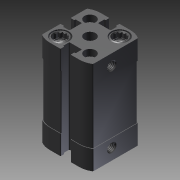
# Autodesk Inventor part: 536203 ADN-15-P---(Z)
Saved by Autodesk Inventor 2011 SP1 (Build 150282100, 282)
## iProperties
Created: 2018-05-28
Part Number: 536203 ADN-15-P---(Z)
Catalog Web Link: www.cadenas.de
Description: ADN-(Z)-Compact cylinder - Z
Vendor: FESTO
Document SubType Name: Modeling
Designer: psAdmin
Manufacturer: FESTO
Mass: 25.558 g
Surface Area: 133.612 cm^2
Volume: 25.558 cm^3
Density: 1 g/cm^3
Category: PARTsolutions
Company: FESTO
Title: 536203 ADN-15-P---(Z)
Author: Cadenas PARTsolutions
Comments: Compact cylinder - Z
PSOL_IDENT_0: {$CADENAS_DATA\23d-libs\festo\parts\a\adn\parts\adn_zr.prj},210 {VTYP=3D},{NB=536203 ADN-15-P---(Z)}
PSOL_IDENT_1: ,{LINA=536203 ADN-15-P---(Z)},{NN=ADN-(Z)},{DATE=06.10.2015 11:54:02},{GEOMDATE=22.09.2015 09:31:00}
PSOL_IDENT_2: ,{VERSION=},{LINEID=5510},{LINESUBID=-1},{WBVAR=HUB,DF,Q,S2S20,S1,R8,TT}  {NB=536203 ADN-15-P---(Z)}
PSOL_IDENT_3: ,{LINA=536203 ADN-15-P---(Z)},{KT=536203},{TNR=536203},{AUSF=ADN},{KDM=12},{BG=17.000},{VERS=1},{HUB
PSOL_IDENT_4: P=-},{HUB=15.00000},{HUB1=[1-300]},{HUB2=-},{HUB3=0},{THC='A','I'},{DF=P},{GA=A},{HUBL=variable},{HU
PSOL_IDENT_5: BC=hubc error},{Q=-},{VAR1C='-','Q'},{S2S20=-},{VAR2C='-','S2'},{VAR5C='-','S6'},{S1=-},{R8=-},{R81='
PSOL_IDENT_6: -'},{TT=-},{TT1='-'},{VAR6C='-'},{VAR7C='-','R3'},{HUBALG=[1-300]},{A=10.000},{A1=0.000},{AF=8.000},
PSOL_IDENT_7: {AF1=0.000},{AF2=8.000},{AF3=0.000},{B=0.000},{B1=0.000},{BG1=0.000},{D1=9.000},{D2=6.000},{D3=32.00
PSOL_IDENT_8: 0},{D4=0.000},{D5=4.000},{D6=M3},{D7=3.000},{D8=0.000},{D9=0.000},{E=27.500},{EE=M5},{EEN=5.000},{EE
PSOL_IDENT_9: 1=-},{J=10.500},{J1=2.000},{J11=2},{J2=0.000},{KF=4-48 UNF-2B},{KF1=-},{KF2=4-45 UNF-2B},{KF3=-},{KK=
PSOL_IDENT_10: 10-32 UNF-2A},{KK1=-},{L1=1.500},{L2=35.000},{L3=2.100},{L4=3.500},{L5=0.000},{L6=46.000},{L7=12.000
PSOL_IDENT_11: },{L8=0.000},{L9=1.500},{L10=0.000},{L11=0.000},{MF=6.000},{MM=6.000},{MM1=0.000},{PL=6.000},{RT=M4}
PSOL_IDENT_12: ,{RTN=4},{RTNK=3.242},{SF=3/16},{SF1=-},{SW=5.500},{TG=16.000},{VD=0.000},{VD1=0.000},{WH=4.200},{WH
PSOL_IDENT_13: 1=0.000},{WL=2.700},{WL1=0.000},{Y1=0.300},{Y2=0.500},{ZJ=39.200},{ZM=43.400},{RU=16.600},{R1=10.350
PSOL_IDENT_14: },{R2=0.600},{RA=0.600},{RB1=5.400},{RB2=6.800},{RT1=3.400},{DSK=6.000},{MDK=5.500},{MK=3.000},{MT=1
PSOL_IDENT_15: .300},{MS=2.500},{RUB=0.200},{KFN=3.000},{KFK=2.459},{B111=9.200},{B11=1.000},{B2=5.000},{B3=8.500},
PSOL_IDENT_16: {B4=3.500},{B5=3.000},{B6=6.000},{B7=17.000},{B8=4.000},{B9=6.000},{B10=7.200},{W=0.400},{S=6.000},{
PSOL_IDENT_17: LA=0.000},{LA1=0.000},{LA2=5.500},{LA3=7.000},{LA31=8.000},{LA4=0.000},{LA5=0.000},{LA6=0.000},{RR=4
PSOL_IDENT_18: .000},{LA7=0.000},{LA8=0.000},{LA9=0.000},{LA10=0.000},{ES=0.000},{SS=0.000},{TS=0.000},{WS=0.000},{
PSOL_IDENT_19: DK=0.000},{KS=0.000},{QN=},{S2N=},{S1S20N=},{R8N=},{TTN=},{DFALG='P'}
NN: ADN-(Z)
NT: Compact cylinder - Z
NB: 536203 ADN-15-P---(Z)
NBSYN: $TNR. $AUSF.-$HUB.-$DF.$QN.$S2N.$S1S20N.$R8N.$TTN.---(Z)
LINA: 536203 ADN-15-P---(Z)
TNR: 536203
AUSF: ADN
KDM: 12
BG: 17.000
HUB: 15.00000
DF: P
GA: A
Q: -
S2S20: -
S1: -
R8: -
TT: -
A: 10.000
A1: 0.000
AF: 8.000
AF1: 0.000
AF2: 8.000
AF3: 0.000
B: 0.000
B1: 0.000
BG1: 0.000
D1: 9.000
D2: 6.000
D3: 32.000
D4: 0.000
D5: 4.000
D6: M3
D7: 3.000
D8: 0.000
D9: 0.000
E: 27.500
EE: M5
EE1: -
J: 10.500
J1: 2.000
J2: 0.000
KF: 4-48 UNF-2B
KF1: -
KF2: 4-45 UNF-2B
KF3: -
KK: 10-32 UNF-2A
KK1: -
L1: 1.500
L2: 35.000
L3: 2.100
L4: 3.500
L5: 0.000
L6: 46.000
L7: 12.000
L8: 0.000
L9: 1.500
L10: 0.000
L11: 0.000
MF: 6.000
MM: 6.000
MM1: 0.000
PL: 6.000
RT: M4
RTNK: 3.242
SF: 3/16
SF1: -
SW: 5.500
TG: 16.000
VD: 0.000
VD1: 0.000
WH: 4.200
WH1: 0.000
WL: 2.700
WL1: 0.000
Y1: 0.300
Y2: 0.500
ZJ: 39.200
ZM: 43.400
RU: 16.600
R1: 10.350
R2: 0.600
RA: 0.600
DSK: 6.000
MDK: 5.500
MK: 3.000
MT: 1.300
MS: 2.500
RUB: 0.200
B111: 9.200
B11: 1.000
B2: 5.000
B3: 8.500
B4: 3.500
B5: 3.000
B6: 6.000
B7: 17.000
B8: 4.000
B9: 6.000
B10: 7.200
W: 0.400
S: 6.000
LA: 0.000
LA1: 0.000
LA2: 5.500
LA3: 7.000
LA31: 8.000
LA4: 0.000
LA5: 0.000
LA6: 0.000
RR: 4.000
LA7: 0.000
LA8: 0.000
LA9: 0.000
LA10: 0.000
ES: 0.000
SS: 0.000
TS: 0.000
WS: 0.000
DK: 0.000
KS: 0.000
SUPPLIER: FESTO
ARTICLENO: 536203 ADN-15-P---(Z)
BOMINFO: 536203 ADN-15-P---(Z)
CREATOR: CADENAS GmbH
Autodesk Inventor part; units mm, degrees
sketch "Sketch_26" plane through (0, 0, 0) normal (0, 0, 1) x (1, 0, 0)
  line L0 (-13.75, -2.5) -> (-13.75, -11.5793)
  arc A0 (-13.75, -11.5793) -> (-13.3272, -12.3141) centre (-12.9, -11.5793) ccw
  arc A1 (-13.3272, -12.3141) -> (-8, -13.75) centre (-8, -3.15) ccw
  line L1 (-8, -13.75) -> (-2.5, -13.75)
  arc A2 (-2.5, -13.75) -> (-2.1, -13.35) centre (-2.5, -13.35) ccw
  line L2 (-2.1, -13.35) -> (-2.1, -11.9)
  arc A3 (-2.1, -11.9) -> (-2.3, -11.7) centre (-2.3, -11.9) ccw
  line L3 (-2.3, -11.7) -> (-2.6, -11.7)
  arc A4 (-2.8, -11.5) -> (-2.6, -11.7) centre (-2.6, -11.5) ccw
  line L4 (-2.8, -11.5) -> (-2.8, -8.7)
  arc A5 (-2.4, -8.3) -> (-2.8, -8.7) centre (-2.4, -8.7) ccw
  line L5 (-2.4, -8.3) -> (3.6, -8.3)
  arc A6 (4, -8.7) -> (3.6, -8.3) centre (3.6, -8.7) ccw
  line L6 (4, -8.7) -> (4, -11.5)
  arc A7 (3.8, -11.7) -> (4, -11.5) centre (3.8, -11.5) ccw
  line L7 (3.8, -11.7) -> (3.5, -11.7)
  arc A8 (3.5, -11.7) -> (3.3, -11.9) centre (3.5, -11.9) ccw
  line L8 (3.3, -11.9) -> (3.3, -13.35)
  arc A9 (3.3, -13.35) -> (3.7, -13.75) centre (3.7, -13.35) ccw
  line L9 (3.7, -13.75) -> (8, -13.75)
  arc A10 (8, -13.75) -> (13.3272, -12.3141) centre (8, -3.15) ccw
  arc A11 (13.3272, -12.3141) -> (13.75, -11.5793) centre (12.9, -11.5793) ccw
  line L10 (13.75, -11.5793) -> (13.75, 11.5793)
  arc A12 (13.75, 11.5793) -> (13.3272, 12.3141) centre (12.9, 11.5793) ccw
  arc A13 (13.3272, 12.3141) -> (8, 13.75) centre (8, 3.15) ccw
  line L11 (8, 13.75) -> (2.5, 13.75)
  arc A14 (2.5, 13.75) -> (2.1, 13.35) centre (2.5, 13.35) ccw
  line L12 (2.1, 13.35) -> (2.1, 11.9)
  arc A15 (2.1, 11.9) -> (2.3, 11.7) centre (2.3, 11.9) ccw
  line L13 (2.3, 11.7) -> (2.6, 11.7)
  arc A16 (2.8, 11.5) -> (2.6, 11.7) centre (2.6, 11.5) ccw
  line L14 (2.8, 11.5) -> (2.8, 8.7)
  arc A17 (2.4, 8.3) -> (2.8, 8.7) centre (2.4, 8.7) ccw
  line L15 (2.4, 8.3) -> (-3.6, 8.3)
  arc A18 (-4, 8.7) -> (-3.6, 8.3) centre (-3.6, 8.7) ccw
  line L16 (-4, 8.7) -> (-4, 11.5)
  arc A19 (-3.8, 11.7) -> (-4, 11.5) centre (-3.8, 11.5) ccw
  line L17 (-3.8, 11.7) -> (-3.5, 11.7)
  arc A20 (-3.5, 11.7) -> (-3.3, 11.9) centre (-3.5, 11.9) ccw
  line L18 (-3.3, 11.9) -> (-3.3, 13.35)
  arc A21 (-3.3, 13.35) -> (-3.7, 13.75) centre (-3.7, 13.35) ccw
  line L19 (-3.7, 13.75) -> (-8, 13.75)
  arc A22 (-8, 13.75) -> (-13.3272, 12.3141) centre (-8, 3.15) ccw
  arc A23 (-13.3272, 12.3141) -> (-13.75, 11.5793) centre (-12.9, 11.5793) ccw
  line L20 (-13.75, 11.5793) -> (-13.75, 3.7)
  arc A24 (-13.75, 3.7) -> (-13.35, 3.3) centre (-13.35, 3.7) ccw
  line L21 (-13.35, 3.3) -> (-11.9, 3.3)
  arc A25 (-11.9, 3.3) -> (-11.7, 3.5) centre (-11.9, 3.5) ccw
  line L22 (-11.7, 3.5) -> (-11.7, 3.8)
  arc A26 (-11.5, 4) -> (-11.7, 3.8) centre (-11.5, 3.8) ccw
  line L23 (-11.5, 4) -> (-8.7, 4)
  arc A27 (-8.3, 3.6) -> (-8.7, 4) centre (-8.7, 3.6) ccw
  line L24 (-8.3, 3.6) -> (-8.3, -2.4)
  arc A28 (-8.7, -2.8) -> (-8.3, -2.4) centre (-8.7, -2.4) ccw
  line L25 (-8.7, -2.8) -> (-11.5, -2.8)
  arc A29 (-11.7, -2.6) -> (-11.5, -2.8) centre (-11.5, -2.6) ccw
  line L26 (-11.7, -2.6) -> (-11.7, -2.3)
  arc A30 (-11.7, -2.3) -> (-11.9, -2.1) centre (-11.9, -2.3) ccw
  line L27 (-11.9, -2.1) -> (-13.35, -2.1)
  arc A31 (-13.35, -2.1) -> (-13.75, -2.5) centre (-13.35, -2.5) ccw
  constraints: 64 point on circle, 56 end point, 32 centre point
extrude "Extrusion1" add sketch "Sketch_26" against normal blind 50
sketch "Sketch_112" plane through (0, 0, -10.5) normal (0, 0, 1) x (1, 0, 0)
  line L0 (-27.5, -27.5) -> (27.5, -27.5)
  line L1 (27.5, -27.5) -> (27.5, 27.5)
  line L2 (27.5, 27.5) -> (-27.5, 27.5)
  line L3 (-27.5, 27.5) -> (-27.5, -27.5)
  line L4 (-13.5, -2.5) -> (-13.5, -11.3293)
  arc A0 (-13.5, -11.3293) -> (-13.0772, -12.0641) centre (-12.65, -11.3293) ccw
  arc A1 (-13.0772, -12.0641) -> (-7.75, -13.5) centre (-7.75, -2.9) ccw
  line L5 (-7.75, -13.5) -> (-2.5, -13.5)
  arc A2 (-2.5, -13.5) -> (-2.1, -13.1) centre (-2.5, -13.1) ccw
  line L6 (-2.1, -13.1) -> (-2.1, -11.85)
  arc A3 (-2.1, -11.85) -> (-2.25, -11.7) centre (-2.25, -11.85) ccw
  line L7 (-2.25, -11.7) -> (-2.6, -11.7)
  arc A4 (-2.8, -11.5) -> (-2.6, -11.7) centre (-2.6, -11.5) ccw
  line L8 (-2.8, -11.5) -> (-2.8, -8.7)
  arc A5 (-2.4, -8.3) -> (-2.8, -8.7) centre (-2.4, -8.7) ccw
  line L9 (-2.4, -8.3) -> (3.6, -8.3)
  arc A6 (4, -8.7) -> (3.6, -8.3) centre (3.6, -8.7) ccw
  line L10 (4, -8.7) -> (4, -11.5)
  arc A7 (3.8, -11.7) -> (4, -11.5) centre (3.8, -11.5) ccw
  line L11 (3.8, -11.7) -> (3.45, -11.7)
  arc A8 (3.45, -11.7) -> (3.3, -11.85) centre (3.45, -11.85) ccw
  line L12 (3.3, -11.85) -> (3.3, -13.1)
  arc A9 (3.3, -13.1) -> (3.7, -13.5) centre (3.7, -13.1) ccw
  line L13 (3.7, -13.5) -> (7.75, -13.5)
  arc A10 (7.75, -13.5) -> (13.0772, -12.0641) centre (7.75, -2.9) ccw
  arc A11 (13.0772, -12.0641) -> (13.5, -11.3293) centre (12.65, -11.3293) ccw
  line L14 (13.5, -11.3293) -> (13.5, 11.3293)
  arc A12 (13.5, 11.3293) -> (13.0772, 12.0641) centre (12.65, 11.3293) ccw
  arc A13 (13.0772, 12.0641) -> (7.75, 13.5) centre (7.75, 2.9) ccw
  line L15 (7.75, 13.5) -> (2.5, 13.5)
  arc A14 (2.5, 13.5) -> (2.1, 13.1) centre (2.5, 13.1) ccw
  line L16 (2.1, 13.1) -> (2.1, 11.85)
  arc A15 (2.1, 11.85) -> (2.25, 11.7) centre (2.25, 11.85) ccw
  line L17 (2.25, 11.7) -> (2.6, 11.7)
  arc A16 (2.8, 11.5) -> (2.6, 11.7) centre (2.6, 11.5) ccw
  line L18 (2.8, 11.5) -> (2.8, 8.7)
  arc A17 (2.4, 8.3) -> (2.8, 8.7) centre (2.4, 8.7) ccw
  line L19 (2.4, 8.3) -> (-3.6, 8.3)
  arc A18 (-4, 8.7) -> (-3.6, 8.3) centre (-3.6, 8.7) ccw
  line L20 (-4, 8.7) -> (-4, 11.5)
  arc A19 (-3.8, 11.7) -> (-4, 11.5) centre (-3.8, 11.5) ccw
  line L21 (-3.8, 11.7) -> (-3.45, 11.7)
  arc A20 (-3.45, 11.7) -> (-3.3, 11.85) centre (-3.45, 11.85) ccw
  line L22 (-3.3, 11.85) -> (-3.3, 13.1)
  arc A21 (-3.3, 13.1) -> (-3.7, 13.5) centre (-3.7, 13.1) ccw
  line L23 (-3.7, 13.5) -> (-7.75, 13.5)
  arc A22 (-7.75, 13.5) -> (-13.0772, 12.0641) centre (-7.75, 2.9) ccw
  arc A23 (-13.0772, 12.0641) -> (-13.5, 11.3293) centre (-12.65, 11.3293) ccw
  line L24 (-13.5, 11.3293) -> (-13.5, 3.7)
  arc A24 (-13.5, 3.7) -> (-13.1, 3.3) centre (-13.1, 3.7) ccw
  line L25 (-13.1, 3.3) -> (-11.85, 3.3)
  arc A25 (-11.85, 3.3) -> (-11.7, 3.45) centre (-11.85, 3.45) ccw
  line L26 (-11.7, 3.45) -> (-11.7, 3.8)
  arc A26 (-11.5, 4) -> (-11.7, 3.8) centre (-11.5, 3.8) ccw
  line L27 (-11.5, 4) -> (-8.7, 4)
  arc A27 (-8.3, 3.6) -> (-8.7, 4) centre (-8.7, 3.6) ccw
  line L28 (-8.3, 3.6) -> (-8.3, -2.4)
  arc A28 (-8.7, -2.8) -> (-8.3, -2.4) centre (-8.7, -2.4) ccw
  line L29 (-8.7, -2.8) -> (-11.5, -2.8)
  arc A29 (-11.7, -2.6) -> (-11.5, -2.8) centre (-11.5, -2.6) ccw
  line L30 (-11.7, -2.6) -> (-11.7, -2.25)
  arc A30 (-11.7, -2.25) -> (-11.85, -2.1) centre (-11.85, -2.25) ccw
  line L31 (-11.85, -2.1) -> (-13.1, -2.1)
  arc A31 (-13.1, -2.1) -> (-13.5, -2.5) centre (-13.1, -2.5) ccw
  constraints: 64 end point, 64 point on circle, 32 centre point
extrude "Extrusion2" cut sketch "Sketch_112" against normal blind 29
sketch "Skizze_3_ALT_Drilling_1" plane through (0, -2, 0) normal (0, 1, 0) x (1, 0, 0)
  line L0 (13.75, 6) -> (6.75, 6)
  line L1 (6.75, 6) -> (6.75, 8.067)
  line L2 (6.75, 8.067) -> (13.317, 8.067)
  line L3 (13.317, 8.067) -> (13.75, 8.5)
  line L4 (13.75, 8.5) -> (13.75, 6)
  line L5 (13.75, 6) -> (6.75, 6)
  constraints: 12 end point
revolve "Revolution1" cut sketch "Skizze_3_ALT_Drilling_1" angle 360 about axis through (13.75, -2, -6) along (1, 0, 0)
thread "Thread1" size "M5x0.8" class "6H" standard "ISO Metric profile" length 5.067
sketch "Skizze_4_ALT_Drilling_2" plane through (0, -2, 0) normal (0, 1, 0) x (1, 0, 0)
  line L0 (13.75, 44) -> (5.75, 44)
  line L1 (5.75, 44) -> (5.75, 46.067)
  line L2 (5.75, 46.067) -> (13.317, 46.067)
  line L3 (13.317, 46.067) -> (13.75, 46.5)
  line L4 (13.75, 46.5) -> (13.75, 44)
  line L5 (13.75, 44) -> (5.75, 44)
  constraints: 12 end point
revolve "Revolution2" cut sketch "Skizze_4_ALT_Drilling_2" angle 360 about axis through (13.75, -2, -44) along (1, 0, 0)
thread "Thread2" size "M5x0.8" class "6H" standard "ISO Metric profile" length 5.067
sketch "Skizze_5_ALT_Drilling_3" plane through (0, 0, 0) normal (1, 0, 0) x (0, 1, 0)
  line L0 (0, -38) -> (0, 1)
  line L1 (0, 1) -> (3, 1)
  line L2 (3, 1) -> (3, -20)
  line L3 (3, -20) -> (6, -20)
  line L4 (6, -20) -> (6, -38)
  line L5 (6, -38) -> (0, -38)
  line L6 (0, -38) -> (0, 1)
  constraints: 14 end point
revolve "Revolution3" cut sketch "Skizze_5_ALT_Drilling_3" angle 360 about axis through (0, 0, -38) along (0, 0, -1)
sketch "Skizze_7_ALT_Drilling_4" plane through (0, 0, 0) normal (1, 0, 0) x (0, 1, 0)
  line L0 (0, -50) -> (0, -47.9)
  line L1 (0, -47.9) -> (4.5, -47.9)
  line L2 (4.5, -47.9) -> (4.5, -50)
  line L3 (4.5, -50) -> (0, -50)
  line L4 (0, -50) -> (0, -47.9)
  constraints: 10 end point
revolve "Revolution4" cut sketch "Skizze_7_ALT_Drilling_4" angle 360 about axis through (0, 0, -50) along (0, 0, -1)
sketch "Skizze_8_ALT_Drilling_5" plane through (8, 0, 0) normal (1, 0, 0) x (0, 0, -1)
  line L0 (17, 8) -> (0, 8)
  line L1 (0, 8) -> (0, 12.6)
  line L2 (0, 12.6) -> (5, 12.6)
  line L3 (5, 12.6) -> (5, 11)
  line L4 (5, 11) -> (17, 11)
  line L5 (17, 11) -> (17, 8)
  line L6 (17, 8) -> (0, 8)
  constraints: 14 end point
revolve "Revolution5" cut sketch "Skizze_8_ALT_Drilling_5" angle 360 about axis through (8, 8, -17) along (0, 0, -1)
sketch "Sketch_27" plane through (8, 0, 0) normal (1, 0, 0) x (0, 0, -1)
  line L0 (17, 8) -> (0, 8)
  line L1 (0, 11.6) -> (1.0392, 11)
  line L2 (1.0392, 11) -> (3.5, 11)
  line L3 (3.5, 11) -> (3.5, 10)
  line L4 (3.5, 10) -> (3.879, 9.621)
  line L5 (3.879, 9.621) -> (17, 9.621)
  line L6 (17, 9.621) -> (17, 12)
  line L7 (17, 12) -> (5, 12)
  line L8 (5, 12) -> (5, 12.25)
  line L9 (5, 12.25) -> (0.4, 12.25)
  line L10 (0.4, 12.25) -> (0, 11.85)
  line L11 (0, 11.85) -> (0, 11.6)
  constraints: 24 end point
revolve "Revolution6" add sketch "Sketch_27" angle 360 about axis through (8, 8, -17) along (0, 0, -1)
thread "Thread3" size "M4x0.7" class "6H" standard "ISO Metric profile" full length
sketch "Sketch_1_ALT_Drilling_6" plane through (8, 0, 0) normal (1, 0, 0) x (0, 0, -1)
  line L0 (50, 8) -> (33, 8)
  line L1 (33, 8) -> (33, 11)
  line L2 (33, 11) -> (45, 11)
  line L3 (45, 11) -> (45, 12.6)
  line L4 (45, 12.6) -> (50, 12.6)
  line L5 (50, 12.6) -> (50, 8)
  line L6 (50, 8) -> (33, 8)
  constraints: 14 end point
revolve "Revolution7" cut sketch "Sketch_1_ALT_Drilling_6" angle 360 about axis through (8, 8, -50) along (0, 0, -1)
sketch "Sketch_86_ALT_Drilling_7" plane through (8, 0, 0) normal (1, 0, 0) x (0, 0, -1)
  line L0 (33, 8) -> (17, 8)
  line L1 (17, 8) -> (17, 10)
  line L2 (17, 10) -> (33, 10)
  line L3 (33, 10) -> (33, 8)
  line L4 (33, 8) -> (17, 8)
  constraints: 10 end point
revolve "Revolution8" cut sketch "Sketch_86_ALT_Drilling_7" angle 360 about axis through (8, 8, -33) along (0, 0, -1)
sketch "Sketch_28" plane through (8, 0, 0) normal (1, 0, 0) x (0, 0, -1)
  line L0 (50, 8) -> (33, 8)
  line L1 (33, 12) -> (33, 9.621)
  line L2 (33, 9.621) -> (46.121, 9.621)
  line L3 (46.121, 9.621) -> (46.5, 10)
  line L4 (46.5, 10) -> (46.5, 11)
  line L5 (46.5, 11) -> (48.9608, 11)
  line L6 (48.9608, 11) -> (50, 11.6)
  line L7 (50, 11.6) -> (50, 11.85)
  line L8 (50, 11.85) -> (49.6, 12.25)
  line L9 (49.6, 12.25) -> (45, 12.25)
  line L10 (45, 12.25) -> (45, 12)
  line L11 (45, 12) -> (33, 12)
  constraints: 24 end point
revolve "Revolution9" add sketch "Sketch_28" angle 360 about axis through (8, 8, -50) along (0, 0, -1)
thread "Thread4" size "M4x0.7" class "6H" standard "ISO Metric profile" full length
sketch "Skizze_9_ALT_Drilling_8" plane through (-8, 0, 0) normal (1, 0, 0) x (0, 0, -1)
  line L0 (25, -8) -> (0, -8)
  line L1 (0, -8) -> (0, -3.4)
  line L2 (0, -3.4) -> (5, -3.4)
  line L3 (5, -3.4) -> (5, -5)
  line L4 (5, -5) -> (17, -5)
  line L5 (17, -5) -> (17, -8)
  line L6 (17, -8) -> (0, -8)
  constraints: 14 end point
revolve "Revolution10" cut sketch "Skizze_9_ALT_Drilling_8" angle 360 about axis through (-8, -8, -25) along (0, 0, -1)
sketch "Sketch_2_ALT_Drilling_9" plane through (-8, 0, 0) normal (1, 0, 0) x (0, 0, -1)
  line L0 (50, -8) -> (33, -8)
  line L1 (33, -8) -> (33, -5)
  line L2 (33, -5) -> (45, -5)
  line L3 (45, -5) -> (45, -3.4)
  line L4 (45, -3.4) -> (50, -3.4)
  line L5 (50, -3.4) -> (50, -8)
  line L6 (50, -8) -> (33, -8)
  constraints: 14 end point
revolve "Revolution11" cut sketch "Sketch_2_ALT_Drilling_9" angle 360 about axis through (-8, -8, -50) along (0, 0, -1)
sketch "Sketch_29" plane through (-8, 0, 0) normal (1, 0, 0) x (0, 0, -1)
  line L0 (17, -8) -> (0, -8)
  line L1 (0, -4.4) -> (1.0392, -5)
  line L2 (1.0392, -5) -> (3.5, -5)
  line L3 (3.5, -5) -> (3.5, -6)
  line L4 (3.5, -6) -> (3.879, -6.379)
  line L5 (3.879, -6.379) -> (17, -6.379)
  line L6 (17, -6.379) -> (17, -4)
  line L7 (17, -4) -> (5, -4)
  line L8 (5, -4) -> (5, -3.75)
  line L9 (5, -3.75) -> (0.4, -3.75)
  line L10 (0.4, -3.75) -> (0, -4.15)
  line L11 (0, -4.15) -> (0, -4.4)
  constraints: 24 end point
revolve "Revolution12" add sketch "Sketch_29" angle 360 about axis through (-8, -8, -17) along (0, 0, -1)
thread "Thread5" size "M4x0.7" class "6H" standard "ISO Metric profile" full length
sketch "Sketch_30" plane through (-8, 0, 0) normal (1, 0, 0) x (0, 0, -1)
  line L0 (50, -8) -> (33, -8)
  line L1 (33, -4) -> (33, -6.379)
  line L2 (33, -6.379) -> (46.121, -6.379)
  line L3 (46.121, -6.379) -> (46.5, -6)
  line L4 (46.5, -6) -> (46.5, -5)
  line L5 (46.5, -5) -> (48.9608, -5)
  line L6 (48.9608, -5) -> (50, -4.4)
  line L7 (50, -4.4) -> (50, -4.15)
  line L8 (50, -4.15) -> (49.6, -3.75)
  line L9 (49.6, -3.75) -> (45, -3.75)
  line L10 (45, -3.75) -> (45, -4)
  line L11 (45, -4) -> (33, -4)
  constraints: 24 end point
revolve "Revolution13" add sketch "Sketch_30" angle 360 about axis through (-8, -8, -50) along (0, 0, -1)
thread "Thread6" size "M4x0.7" class "6H" standard "ISO Metric profile" full length
sketch "Skizze_12_ALT_Drilling_10" plane through (8, 0, 0) normal (1, 0, 0) x (0, 0, -1)
  line L0 (33, -8) -> (-0.1, -8)
  line L1 (-0.1, -8) -> (-0.1, -5)
  line L2 (-0.1, -5) -> (3.5, -5)
  line L3 (3.5, -5) -> (3.5, -6)
  line L4 (3.5, -6) -> (3.879, -6.379)
  line L5 (3.879, -6.379) -> (33, -6.379)
  line L6 (33, -6.379) -> (33, -8)
  line L7 (33, -8) -> (-0.1, -8)
  constraints: 16 end point
revolve "Revolution14" cut sketch "Skizze_12_ALT_Drilling_10" angle 360 about axis through (8, -8, -33) along (0, 0, -1)
thread "Thread7" size "M4x0.7" class "6H" standard "ISO Metric profile" length 6.621
sketch "Sketch_123" plane through (8, 0, 0) normal (1, 0, 0) x (0, 0, -1)
  line L0 (33, -8) -> (10.5, -8)
  line L1 (10.5, -8) -> (10.5, -4)
  line L2 (10.5, -4) -> (33, -4)
  line L3 (33, -4) -> (33, -8)
  line L4 (33, -8) -> (10.5, -8)
  constraints: 10 end point
revolve "Revolution15" add sketch "Sketch_123" angle 360 about axis through (8, -8, -33) along (0, 0, -1)
sketch "Sketch_124_ALT_Drilling_11" plane through (8, 0, 0) normal (1, 0, 0) x (0, 0, -1)
  line L0 (33, -8) -> (10.5, -8)
  line L1 (10.5, -8) -> (10.5, -6)
  line L2 (10.5, -6) -> (33, -6)
  line L3 (33, -6) -> (33, -8)
  line L4 (33, -8) -> (10.5, -8)
  constraints: 10 end point
revolve "Revolution16" cut sketch "Sketch_124_ALT_Drilling_11" angle 360 about axis through (8, -8, -33) along (0, 0, -1)
sketch "Sketch_3_ALT_Drilling_12" plane through (8, 0, 0) normal (1, 0, 0) x (0, 0, -1)
  line L0 (50.1, -8) -> (25, -8)
  line L1 (25, -8) -> (25, -6.379)
  line L2 (25, -6.379) -> (46.121, -6.379)
  line L3 (46.121, -6.379) -> (46.5, -6)
  line L4 (46.5, -6) -> (46.5, -5)
  line L5 (46.5, -5) -> (50.1, -5)
  line L6 (50.1, -5) -> (50.1, -8)
  line L7 (50.1, -8) -> (25, -8)
  constraints: 16 end point
revolve "Revolution17" cut sketch "Sketch_3_ALT_Drilling_12" angle 360 about axis through (8, -8, -50.1) along (0, 0, -1)
thread "Thread8" size "M4x0.7" class "6H" standard "ISO Metric profile" length 6.621
sketch "Sketch_117" plane through (8, 0, 0) normal (1, 0, 0) x (0, 0, -1)
  line L0 (39.5, -8) -> (17, -8)
  line L1 (17, -8) -> (17, -4)
  line L2 (17, -4) -> (39.5, -4)
  line L3 (39.5, -4) -> (39.5, -8)
  line L4 (39.5, -8) -> (17, -8)
  constraints: 10 end point
revolve "Revolution18" add sketch "Sketch_117" angle 360 about axis through (8, -8, -39.5) along (0, 0, -1)
sketch "Sketch_119_ALT_Drilling_13" plane through (8, 0, 0) normal (1, 0, 0) x (0, 0, -1)
  line L0 (39.5, -8) -> (17, -8)
  line L1 (17, -8) -> (17, -6)
  line L2 (17, -6) -> (39.5, -6)
  line L3 (39.5, -6) -> (39.5, -8)
  line L4 (39.5, -8) -> (17, -8)
  constraints: 10 end point
revolve "Revolution19" cut sketch "Sketch_119_ALT_Drilling_13" angle 360 about axis through (8, -8, -39.5) along (0, 0, -1)
sketch "Skizze_13_ALT_Drilling_14" plane through (-8, 0, 0) normal (1, 0, 0) x (0, 0, -1)
  line L0 (33, 8) -> (-0.1, 8)
  line L1 (-0.1, 8) -> (-0.1, 11)
  line L2 (-0.1, 11) -> (3.5, 11)
  line L3 (3.5, 11) -> (3.5, 10)
  line L4 (3.5, 10) -> (3.879, 9.621)
  line L5 (3.879, 9.621) -> (33, 9.621)
  line L6 (33, 9.621) -> (33, 8)
  line L7 (33, 8) -> (-0.1, 8)
  constraints: 16 end point
revolve "Revolution20" cut sketch "Skizze_13_ALT_Drilling_14" angle 360 about axis through (-8, 8, -33) along (0, 0, -1)
thread "Thread9" size "M4x0.7" class "6H" standard "ISO Metric profile" length 6.621
sketch "Sketch_121" plane through (-8, 0, 0) normal (1, 0, 0) x (0, 0, -1)
  line L0 (33, 8) -> (10.5, 8)
  line L1 (10.5, 8) -> (10.5, 12)
  line L2 (10.5, 12) -> (33, 12)
  line L3 (33, 12) -> (33, 8)
  line L4 (33, 8) -> (10.5, 8)
  constraints: 10 end point
revolve "Revolution21" add sketch "Sketch_121" angle 360 about axis through (-8, 8, -33) along (0, 0, -1)
sketch "Sketch_122_ALT_Drilling_15" plane through (-8, 0, 0) normal (1, 0, 0) x (0, 0, -1)
  line L0 (33, 8) -> (10.5, 8)
  line L1 (10.5, 8) -> (10.5, 10)
  line L2 (10.5, 10) -> (33, 10)
  line L3 (33, 10) -> (33, 8)
  line L4 (33, 8) -> (10.5, 8)
  constraints: 10 end point
revolve "Revolution22" cut sketch "Sketch_122_ALT_Drilling_15" angle 360 about axis through (-8, 8, -33) along (0, 0, -1)
sketch "Sketch_4_ALT_Drilling_16" plane through (-8, 0, 0) normal (1, 0, 0) x (0, 0, -1)
  line L0 (50.1, 8) -> (25, 8)
  line L1 (25, 8) -> (25, 9.621)
  line L2 (25, 9.621) -> (46.121, 9.621)
  line L3 (46.121, 9.621) -> (46.5, 10)
  line L4 (46.5, 10) -> (46.5, 11)
  line L5 (46.5, 11) -> (50.1, 11)
  line L6 (50.1, 11) -> (50.1, 8)
  line L7 (50.1, 8) -> (25, 8)
  constraints: 16 end point
revolve "Revolution23" cut sketch "Sketch_4_ALT_Drilling_16" angle 360 about axis through (-8, 8, -50.1) along (0, 0, -1)
thread "Thread10" size "M4x0.7" class "6H" standard "ISO Metric profile" length 6.621
sketch "Sketch_118" plane through (-8, 0, 0) normal (1, 0, 0) x (0, 0, -1)
  line L0 (39.5, 8) -> (17, 8)
  line L1 (17, 8) -> (17, 12)
  line L2 (17, 12) -> (39.5, 12)
  line L3 (39.5, 12) -> (39.5, 8)
  line L4 (39.5, 8) -> (17, 8)
  constraints: 10 end point
revolve "Revolution24" add sketch "Sketch_118" angle 360 about axis through (-8, 8, -39.5) along (0, 0, -1)
sketch "Sketch_120_ALT_Drilling_17" plane through (-8, 0, 0) normal (1, 0, 0) x (0, 0, -1)
  line L0 (39.5, 8) -> (17, 8)
  line L1 (17, 8) -> (17, 10)
  line L2 (17, 10) -> (39.5, 10)
  line L3 (39.5, 10) -> (39.5, 8)
  line L4 (39.5, 8) -> (17, 8)
  constraints: 10 end point
revolve "Revolution25" cut sketch "Sketch_120_ALT_Drilling_17" angle 360 about axis through (-8, 8, -39.5) along (0, 0, -1)
sketch "Sketch_85_ALT_Drilling_18" plane through (-8, 0, 0) normal (1, 0, 0) x (0, 0, -1)
  line L0 (33, -8) -> (17, -8)
  line L1 (17, -8) -> (17, -6)
  line L2 (17, -6) -> (33, -6)
  line L3 (33, -6) -> (33, -8)
  line L4 (33, -8) -> (17, -8)
  constraints: 10 end point
revolve "Revolution26" cut sketch "Sketch_85_ALT_Drilling_18" angle 360 about axis through (-8, -8, -33) along (0, 0, -1)
sketch "Sketch_8" plane through (0, 0, 0) normal (0, 0, 1) x (1, 0, 0)
  line L0 (-11.4641, -8) -> (-11, -8.8038)
  line L1 (-11, -8.8038) -> (-11, -9.7321)
  line L2 (-11, -9.7321) -> (-10.1962, -10.1962)
  line L3 (-10.1962, -10.1962) -> (-9.7321, -11)
  line L4 (-9.7321, -11) -> (-8.8038, -11)
  line L5 (-8.8038, -11) -> (-8, -11.4641)
  line L6 (-8, -11.4641) -> (-7.1962, -11)
  line L7 (-7.1962, -11) -> (-6.2679, -11)
  line L8 (-6.2679, -11) -> (-5.8038, -10.1962)
  line L9 (-5.8038, -10.1962) -> (-5, -9.7321)
  line L10 (-5, -9.7321) -> (-5, -8.8038)
  line L11 (-5, -8.8038) -> (-4.5359, -8)
  line L12 (-4.5359, -8) -> (-5, -7.1962)
  line L13 (-5, -7.1962) -> (-5, -6.2679)
  line L14 (-5, -6.2679) -> (-5.8038, -5.8038)
  line L15 (-5.8038, -5.8038) -> (-6.2679, -5)
  line L16 (-6.2679, -5) -> (-7.1962, -5)
  line L17 (-7.1962, -5) -> (-8, -4.5359)
  line L18 (-8, -4.5359) -> (-8.8038, -5)
  line L19 (-8.8038, -5) -> (-9.7321, -5)
  line L20 (-9.7321, -5) -> (-10.1962, -5.8038)
  line L21 (-10.1962, -5.8038) -> (-11, -6.2679)
  line L22 (-11, -6.2679) -> (-11, -7.1962)
  line L23 (-11, -7.1962) -> (-11.4641, -8)
  constraints: 48 end point
extrude "Extrusion3" cut sketch "Sketch_8" against normal blind 3
sketch "Sketch_7" plane through (0, 0, 0) normal (0, 0, 1) x (1, 0, 0)
  line L0 (4.5359, 8) -> (5, 7.1962)
  line L1 (5, 7.1962) -> (5, 6.2679)
  line L2 (5, 6.2679) -> (5.8038, 5.8038)
  line L3 (5.8038, 5.8038) -> (6.2679, 5)
  line L4 (6.2679, 5) -> (7.1962, 5)
  line L5 (7.1962, 5) -> (8, 4.5359)
  line L6 (8, 4.5359) -> (8.8038, 5)
  line L7 (8.8038, 5) -> (9.7321, 5)
  line L8 (9.7321, 5) -> (10.1962, 5.8038)
  line L9 (10.1962, 5.8038) -> (11, 6.2679)
  line L10 (11, 6.2679) -> (11, 7.1962)
  line L11 (11, 7.1962) -> (11.4641, 8)
  line L12 (11.4641, 8) -> (11, 8.8038)
  line L13 (11, 8.8038) -> (11, 9.7321)
  line L14 (11, 9.7321) -> (10.1962, 10.1962)
  line L15 (10.1962, 10.1962) -> (9.7321, 11)
  line L16 (9.7321, 11) -> (8.8038, 11)
  line L17 (8.8038, 11) -> (8, 11.4641)
  line L18 (8, 11.4641) -> (7.1962, 11)
  line L19 (7.1962, 11) -> (6.2679, 11)
  line L20 (6.2679, 11) -> (5.8038, 10.1962)
  line L21 (5.8038, 10.1962) -> (5, 9.7321)
  line L22 (5, 9.7321) -> (5, 8.8038)
  line L23 (5, 8.8038) -> (4.5359, 8)
  constraints: 48 end point
extrude "Extrusion4" cut sketch "Sketch_7" against normal blind 3
sketch "Sketch_9" plane through (0, 0, -50) normal (0, 0, 1) x (1, 0, 0)
  line L0 (-11.4641, -8) -> (-11, -8.8038)
  line L1 (-11, -8.8038) -> (-11, -9.7321)
  line L2 (-11, -9.7321) -> (-10.1962, -10.1962)
  line L3 (-10.1962, -10.1962) -> (-9.7321, -11)
  line L4 (-9.7321, -11) -> (-8.8038, -11)
  line L5 (-8.8038, -11) -> (-8, -11.4641)
  line L6 (-8, -11.4641) -> (-7.1962, -11)
  line L7 (-7.1962, -11) -> (-6.2679, -11)
  line L8 (-6.2679, -11) -> (-5.8038, -10.1962)
  line L9 (-5.8038, -10.1962) -> (-5, -9.7321)
  line L10 (-5, -9.7321) -> (-5, -8.8038)
  line L11 (-5, -8.8038) -> (-4.5359, -8)
  line L12 (-4.5359, -8) -> (-5, -7.1962)
  line L13 (-5, -7.1962) -> (-5, -6.2679)
  line L14 (-5, -6.2679) -> (-5.8038, -5.8038)
  line L15 (-5.8038, -5.8038) -> (-6.2679, -5)
  line L16 (-6.2679, -5) -> (-7.1962, -5)
  line L17 (-7.1962, -5) -> (-8, -4.5359)
  line L18 (-8, -4.5359) -> (-8.8038, -5)
  line L19 (-8.8038, -5) -> (-9.7321, -5)
  line L20 (-9.7321, -5) -> (-10.1962, -5.8038)
  line L21 (-10.1962, -5.8038) -> (-11, -6.2679)
  line L22 (-11, -6.2679) -> (-11, -7.1962)
  line L23 (-11, -7.1962) -> (-11.4641, -8)
  constraints: 48 end point
extrude "Extrusion5" cut sketch "Sketch_9" along normal blind 3
sketch "Sketch_10" plane through (0, 0, -50) normal (0, 0, 1) x (1, 0, 0)
  line L0 (4.5359, 8) -> (5, 7.1962)
  line L1 (5, 7.1962) -> (5, 6.2679)
  line L2 (5, 6.2679) -> (5.8038, 5.8038)
  line L3 (5.8038, 5.8038) -> (6.2679, 5)
  line L4 (6.2679, 5) -> (7.1962, 5)
  line L5 (7.1962, 5) -> (8, 4.5359)
  line L6 (8, 4.5359) -> (8.8038, 5)
  line L7 (8.8038, 5) -> (9.7321, 5)
  line L8 (9.7321, 5) -> (10.1962, 5.8038)
  line L9 (10.1962, 5.8038) -> (11, 6.2679)
  line L10 (11, 6.2679) -> (11, 7.1962)
  line L11 (11, 7.1962) -> (11.4641, 8)
  line L12 (11.4641, 8) -> (11, 8.8038)
  line L13 (11, 8.8038) -> (11, 9.7321)
  line L14 (11, 9.7321) -> (10.1962, 10.1962)
  line L15 (10.1962, 10.1962) -> (9.7321, 11)
  line L16 (9.7321, 11) -> (8.8038, 11)
  line L17 (8.8038, 11) -> (8, 11.4641)
  line L18 (8, 11.4641) -> (7.1962, 11)
  line L19 (7.1962, 11) -> (6.2679, 11)
  line L20 (6.2679, 11) -> (5.8038, 10.1962)
  line L21 (5.8038, 10.1962) -> (5, 9.7321)
  line L22 (5, 9.7321) -> (5, 8.8038)
  line L23 (5, 8.8038) -> (4.5359, 8)
  constraints: 48 end point
extrude "Extrusion6" cut sketch "Sketch_10" along normal blind 3
ref_plane "CYLINDER_XY" through (0, 0, -38) normal (0, 0, 1) x (1, 0, 0)
ref_plane "CYLINDER_YZ" through (0, 0, -38) normal (1, 0, 0) x (0, 1, 0)
ref_plane "CYLINDER_ZX" through (0, 0, -38) normal (0, 1, 0) x (0, 0, 1)
ref_plane "FDT_FRONT_XY" through (0, 0, 0) normal (0, 0, 1) x (0, -1, 0)
ref_plane "FDT_FRONT_YZ" through (0, 0, 0) normal (0, -1, 0) x (1, 0, 0)
ref_plane "FDT_FRONT_ZX" through (0, 0, 0) normal (1, 0, 0) x (0, 0, 1)
ref_plane "FDT_QSFRONT_XY" through (13.75, -2, -6) normal (1, 0, 0) x (0, -1, 0)
ref_plane "FDT_QSFRONT_YZ" through (13.75, -2, -6) normal (0, -1, 0) x (0, 0, -1)
ref_plane "FDT_QSFRONT_ZX" through (13.75, -2, -6) normal (0, 0, -1) x (1, 0, 0)
ref_plane "FDT_QSREAR_XY" through (13.75, -2, -44) normal (1, 0, 0) x (0, -1, 0)
ref_plane "FDT_QSREAR_YZ" through (13.75, -2, -44) normal (0, -1, 0) x (0, 0, -1)
ref_plane "FDT_QSREAR_ZX" through (13.75, -2, -44) normal (0, 0, -1) x (1, 0, 0)
ref_plane "FDT_REAR_XY" through (0, 0, -50) normal (0, 0, 1) x (0, -1, 0)
ref_plane "FDT_REAR_YZ" through (0, 0, -50) normal (0, -1, 0) x (1, 0, 0)
ref_plane "FDT_REAR_ZX" through (0, 0, -50) normal (1, 0, 0) x (0, 0, 1)
ref_plane "FDT_SLOT3_1_XY" through (-0.6, 8.3, -25) normal (0, 1, 0) x (1, 0, 0)
ref_plane "FDT_SLOT3_1_YZ" through (-0.6, 8.3, -25) normal (1, 0, 0) x (0, 0, -1)
ref_plane "FDT_SLOT3_1_ZX" through (-0.6, 8.3, -25) normal (0, 0, -1) x (0, 1, 0)
ref_plane "FDT_SLOT5_1_XY" through (-8.3, 0.6, -25) normal (-1, 0, 0) x (0, 1, 0)
ref_plane "FDT_SLOT5_1_YZ" through (-8.3, 0.6, -25) normal (0, 1, 0) x (0, 0, -1)
ref_plane "FDT_SLOT5_1_ZX" through (-8.3, 0.6, -25) normal (0, 0, -1) x (-1, 0, 0)
ref_plane "FDT_SLOT7_1_XY" through (0.6, -8.3, -25) normal (0, -1, 0) x (-1, 0, 0)
ref_plane "FDT_SLOT7_1_YZ" through (0.6, -8.3, -25) normal (-1, 0, 0) x (0, 0, -1)
ref_plane "FDT_SLOT7_1_ZX" through (0.6, -8.3, -25) normal (0, 0, -1) x (0, -1, 0)
ref_plane "TO_DUMMY_XY" through (0, 0, 0) normal (0, 0, 1) x (1, 0, 0)
ref_plane "TO_DUMMY_YZ" through (0, 0, 0) normal (1, 0, 0) x (0, 1, 0)
ref_plane "TO_DUMMY_ZX" through (0, 0, 0) normal (0, 1, 0) x (0, 0, 1)
body "Solid1"
